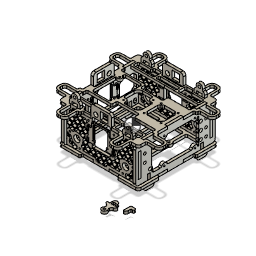
v110 (Autodesk Fusion 360 design; units mm, degrees)
Autodesk Fusion 360 part; units mm, degrees
note: some values were not read from the file. Set by a fixed rule: which sketch regions a step uses.
(part 1 of 3)
sketch "Schizzo1" plane through (0, 0, 0) normal (0, 1, 0) x (1, 0, 0)
  line L0 (-131, 140) -> (-131, 145)
  line L1 (-131, 145) -> (-111, 145)
  line L2 (-111, 140) -> (-131, 140)
  line L3 (-111, 145) -> (-111, 140)
  line L4 (-86, 145) -> (-86, 140)
  line L5 (-86, 140) -> (-71, 140)
  line L6 (-106, 147) -> (-106, 148)
  line L7 (-141, 150) -> (-108, 150)
  arc A0 (-106, 147) -> (-104, 145) centre (-104, 147) ccw
  arc A1 (-106, 148) -> (-108, 150) centre (-108, 148) ccw
  line L8 (25, 10) -> (25, 5)
  line L9 (30, 0) -> (57.5, 0)
  arc A2 (25, 5) -> (30, 0) centre (30, 5) ccw
  arc A3 (-141, 150) -> (-146, 145) centre (-141, 145) ccw
  line L10 (25, 15) -> (20, 15)
  line L11 (20, 35) -> (25, 35)
  line L12 (25, 60) -> (20, 60)
  line L13 (20, 60) -> (20, 75)
  line L14 (25, 10) -> (25, 15)
  line L15 (25, 35) -> (25, 60)
  line L16 (-141, 90) -> (-136, 90)
  line L17 (-136, 90) -> (-136, 75)
  line L18 (-143, 110) -> (-144, 110)
  line L19 (-146, 112) -> (-146, 145)
  arc A4 (-146, 112) -> (-144, 110) centre (-144, 112) ccw
  arc A5 (-141, 108) -> (-143, 110) centre (-143, 108) ccw
  line L20 (-141, 115) -> (-136, 115)
  line L21 (-136, 115) -> (-136, 135)
  line L22 (-136, 135) -> (-141, 135)
  line L23 (-141, 135) -> (-141, 115)
  arc A6 (-108, 0) -> (-106, 2) centre (-108, 2) ccw
  line L24 (-106, 3) -> (-106, 2)
  arc A7 (-104, 5) -> (-106, 3) centre (-104, 3) ccw
  line L25 (-86, 5) -> (-86, 10)
  line L26 (-86, 10) -> (-71, 10)
  line L27 (-136, 60) -> (-136, 75)
  line L28 (-141, 60) -> (-136, 60)
  arc A8 (-143, 40) -> (-141, 42) centre (-143, 42) ccw
  line L29 (-143, 40) -> (-144, 40)
  arc A9 (-144, 40) -> (-146, 38) centre (-144, 38) ccw
  line L30 (-146, 38) -> (-146, 5)
  arc A10 (-146, 5) -> (-141, 0) centre (-141, 5) ccw
  line L31 (-141, 0) -> (-108, 0)
  line L32 (-111, 10) -> (-131, 10)
  line L33 (-131, 10) -> (-131, 5)
  line L34 (-111, 5) -> (-111, 10)
  line L35 (-131, 5) -> (-111, 5)
  line L36 (-141, 15) -> (-141, 35)
  line L37 (-141, 35) -> (-136, 35)
  line L38 (-136, 15) -> (-141, 15)
  line L39 (-136, 35) -> (-136, 15)
  arc A11 (1, 110) -> (-1, 108) centre (1, 108) ccw
  line L40 (1, 110) -> (2, 110)
  arc A12 (2, 110) -> (4, 112) centre (2, 112) ccw
  line L41 (4, 112) -> (4, 145)
  arc A13 (4, 145) -> (-1, 150) centre (-1, 145) ccw
  line L42 (-1, 150) -> (-34, 150)
  arc A14 (-34, 150) -> (-36, 148) centre (-34, 148) ccw
  line L43 (-36, 147) -> (-36, 148)
  arc A15 (-38, 145) -> (-36, 147) centre (-38, 147) ccw
  line L44 (-56, 145) -> (-56, 140)
  line L45 (-56, 140) -> (-71, 140)
  line L46 (-31, 140) -> (-11, 140)
  line L47 (-11, 140) -> (-11, 145)
  line L48 (-31, 145) -> (-31, 140)
  line L49 (-11, 145) -> (-31, 145)
  line L50 (-1, 135) -> (-1, 115)
  line L51 (-1, 115) -> (-6, 115)
  line L52 (-6, 135) -> (-1, 135)
  line L53 (-6, 115) -> (-6, 135)
  line L54 (-1, 90) -> (-6, 90)
  line L55 (-6, 90) -> (-6, 75)
  line L56 (-1, 60) -> (-6, 60)
  line L57 (-6, 60) -> (-6, 75)
  line L58 (-56, 5) -> (-56, 10)
  line L59 (-56, 10) -> (-71, 10)
  arc A16 (-1, 42) -> (1, 40) centre (1, 42) ccw
  line L60 (1, 40) -> (2, 40)
  arc A17 (4, 38) -> (2, 40) centre (2, 38) ccw
  line L61 (4, 38) -> (4, 5)
  arc A18 (-1, 0) -> (4, 5) centre (-1, 5) ccw
  line L62 (-1, 0) -> (-34, 0)
  arc A19 (-36, 2) -> (-34, 0) centre (-34, 2) ccw
  line L63 (-36, 3) -> (-36, 2)
  arc A20 (-36, 3) -> (-38, 5) centre (-38, 3) ccw
  line L64 (-11, 10) -> (-11, 5)
  line L65 (-11, 5) -> (-31, 5)
  line L66 (-31, 10) -> (-11, 10)
  line L67 (-31, 5) -> (-31, 10)
  line L68 (-1, 15) -> (-1, 35)
  line L69 (-1, 35) -> (-6, 35)
  line L70 (-6, 15) -> (-1, 15)
  line L71 (-6, 35) -> (-6, 15)
  line L72 (-231.9997, 2.9999) -> (-231.9997, 2.0006)
  line L73 (-192, 38) -> (-192, 37.0001)
  line L74 (-307, 5) -> (-307, 10)
  line L75 (-197, 60) -> (-202, 60)
  arc A21 (-300, 5) -> (-302, 3) centre (-300, 3) ccw
  arc A22 (-304, 0) -> (-302, 2) centre (-304, 2) ccw
  arc A23 (-197, -0.0001) -> (-192, 4.9999) centre (-197, 4.9999) ccw
  arc A24 (-197, 42) -> (-195, 40) centre (-195, 42) ccw
  arc A25 (-342.0001, 5) -> (-337, 0) centre (-337, 5) ccw
  line L76 (-302, 3) -> (-302, 2)
  line L77 (-195, 40) -> (-194, 40)
  arc A26 (-340, 40) -> (-342, 38) centre (-340, 38) ccw
  arc A27 (-192, 38) -> (-194, 40) centre (-194, 38) ccw
  line L78 (-339, 40) -> (-340, 40)
  line L79 (-202, 60) -> (-202, 75)
  arc A28 (-339, 40) -> (-337, 42) centre (-339, 42) ccw
  arc A29 (-231.9997, 2.9999) -> (-233.9999, 5.0001) centre (-233.9999, 2.9999) ccw
  arc A30 (-231.9997, 2.0006) -> (-229.999, -0.0001) centre (-229.999, 2.0006) ccw
  line L80 (85, 0) -> (57.5, 0)
  arc A31 (85, 0) -> (90, 5) centre (85, 5) ccw
  line L81 (90, 35) -> (90, 60)
  line L82 (90, 60) -> (95, 60)
  line L83 (95, 60) -> (95, 75)
  line L84 (20, 115) -> (25, 115)
  line L85 (25, 115) -> (25, 90)
  line L86 (25, 90) -> (20, 90)
  line L87 (20, 90) -> (20, 75)
  line L88 (25, 140) -> (25, 145)
  line L89 (30, 150) -> (57.5, 150)
  arc A32 (30, 150) -> (25, 145) centre (30, 145) ccw
  line L90 (25, 135) -> (20, 135)
  line L91 (25, 140) -> (25, 135)
  line L92 (57.5, 140) -> (35, 140)
  line L93 (35, 145) -> (35, 140)
  line L94 (57.5, 145) -> (35, 145)
  line L95 (80, 145) -> (80, 140)
  line L96 (80, 140) -> (57.5, 140)
  line L97 (57.5, 145) -> (80, 145)
  arc A33 (90, 145) -> (85, 150) centre (85, 145) ccw
  line L98 (85, 150) -> (57.5, 150)
  line L99 (90, 90) -> (95, 90)
  line L100 (95, 90) -> (95, 75)
  line L101 (-280.5, -113.5) -> (-265.5, -113.5)
  line L102 (-250.5, -113.5) -> (-265.5, -113.5)
  line L103 (-305.5, -113.5) -> (-305.5, -118.5)
  line L104 (-195.5, -98.5) -> (-200.5, -98.5)
  line L105 (-225.5, -43.5) -> (-246, -43.5)
  line L106 (-340.5, -103.5) -> (-340.5, -76)
  line L107 (-251, -18.5) -> (-265.5, -18.5)
  line L108 (-330.5, -108.5) -> (-335.5, -108.5)
  line L109 (-305.5, -38.5) -> (-305.5, -43.5)
  line L110 (-280, -18.5) -> (-265.5, -18.5)
  line L111 (-225.5, -108.5) -> (-250.5, -108.5)
  arc A34 (-340.5, -103.5) -> (-335.5, -108.5) centre (-335.5, -103.5) ccw
  line L112 (-285, -43.5) -> (-285, -23.5)
  line L113 (-330.5, -43.5) -> (-325.5, -43.5)
  line L114 (-305.5, -108.5) -> (-280.5, -108.5)
  line L115 (-325.5, -43.5) -> (-325.5, -38.5)
  line L116 (-330.5, -43.5) -> (-335.5, -43.5)
  line L117 (-305.5, -113.5) -> (-305.5, -108.5)
  line L118 (-200.5, -43.5) -> (-195.5, -43.5)
  line L119 (-195.5, -53.5) -> (-200.5, -53.5)
  line L120 (-589.5, -1.5) -> (-589.5, -1.5)
  line L121 (-320.5, -123.5) -> (-310.5, -123.5)
  arc A35 (-310.5, -123.5) -> (-305.5, -118.5) centre (-310.5, -118.5) ccw
  arc A36 (-325.5, -118.5) -> (-320.5, -123.5) centre (-320.5, -118.5) ccw
  line L122 (-195.5, -76) -> (-195.5, -98.5)
  arc A37 (-335.5, -43.5) -> (-340.5, -48.5) centre (-335.5, -48.5) ccw
  line L123 (-200.5, -108.5) -> (-195.5, -108.5)
  line L124 (-200.5, -43.5) -> (-205.5, -43.5)
  line L125 (-330.5, -108.5) -> (-325.5, -108.5)
  line L126 (-305.5, -43.5) -> (-285, -43.5)
  line L127 (-190.5, -48.5) -> (-190.5, -76)
  line L128 (-225.5, -38.5) -> (-225.5, -43.5)
  line L129 (-200.5, -108.5) -> (-205.5, -108.5)
  line L130 (-340.5, -48.5) -> (-340.5, -76)
  line L131 (-246, -43.5) -> (-246, -23.5)
  arc A38 (-190.5, -48.5) -> (-195.5, -43.5) centre (-195.5, -48.5) ccw
  line L132 (-195.5, -76) -> (-195.5, -53.5)
  line L133 (-190.5, -103.5) -> (-190.5, -76)
  line L134 (-205.5, -43.5) -> (-205.5, -38.5)
  line L135 (-280.5, -108.5) -> (-280.5, -113.5)
  line L136 (-250.5, -108.5) -> (-250.5, -113.5)
  arc A39 (-195.5, -108.5) -> (-190.5, -103.5) centre (-195.5, -103.5) ccw
  arc A40 (-280, -18.5) -> (-285, -23.5) centre (-280, -23.5) ccw
  arc A41 (-246, -23.5) -> (-251, -18.5) centre (-251, -23.5) ccw
  circle A42 centre (-252.9, 89.1) radius 1.25
  circle A43 centre (-281.1, 60.9) radius 1.25
  line L137 (-252.9, 84.1) -> (-250.5, 84.1)
  line L138 (-257.9, 89.1) -> (-257.9, 91.5)
  line L139 (-281.1, 65.9) -> (-283.5, 65.9)
  line L140 (-276.1, 60.9) -> (-276.1, 58.5)
  arc A44 (-257.9, 89.1) -> (-252.9, 84.1) centre (-252.9, 89.1) ccw
  arc A45 (-276.1, 60.9) -> (-281.1, 65.9) centre (-281.1, 60.9) ccw
  arc A46 (-248, 81.6) -> (-250.5, 84.1) centre (-250.5, 81.6) ccw
  arc A47 (-257.9, 91.5) -> (-260.4, 94) centre (-260.4, 91.5) ccw
  arc A48 (-286, 68.4) -> (-283.5, 65.9) centre (-283.5, 68.4) ccw
  arc A49 (-276.1, 58.5) -> (-273.6, 56) centre (-273.6, 58.5) ccw
  line L141 (-31, 140) -> (-25, 140)
  line L142 (-337, 42) -> (-337, 55.5)
  line L143 (-300, 5) -> (-286.5, 5)
  line L144 (-247.5, 5.0001) -> (-233.9999, 5.0001)
  circle A50 centre (33, 54) radius 1.5
  circle A51 centre (33, 112) radius 1.5
  circle A52 centre (-115.5198, -118.5231) radius 1.5
  circle A53 centre (-134.2581, -99.7848) radius 1.5
  circle A54 centre (-120.8585, -105.1234) radius 6
  circle A55 centre (-98.9028, -64.4294) radius 1.5
  line L145 (-82.3205, -124) -> (-80, -124)
  line L146 (-85, -121) -> (-85, -122)
  line L147 (-132, -119) -> (-133, -119)
  line L148 (-135, -117) -> (-135, -116)
  line L149 (-130, -61) -> (-130, -62)
  line L150 (-120, -62) -> (-120, -61)
  line L151 (-80, -124) -> (-77.6795, -124)
  line L152 (-75, -114) -> (-79.3301, -116.5)
  line L153 (-79.3301, -116.5) -> (-79.3301, -121.5)
  line L154 (-79.3301, -121.5) -> (-75, -124)
  arc A56 (-85, -121) -> (-87, -119) centre (-87, -121) ccw
  arc A57 (-85, -122) -> (-84.2458, -123.5646) centre (-83, -122) ccw
  arc A58 (-135, -117) -> (-133, -119) centre (-133, -117) ccw
  arc A59 (-135, -116) -> (-135.7542, -114.4354) centre (-137, -116) ccw
  arc A60 (-130.6699, -119.5064) -> (-132, -119) centre (-132, -121) ccw
  arc A61 (-128, -59) -> (-130, -61) centre (-128, -61) ccw
  arc A62 (-120, -61) -> (-122, -59) centre (-122, -61) ccw
  arc A63 (-103.7753, -65.5513) -> (-105.7243, -64) centre (-105.7243, -66) ccw
  line L155 (-75, -114) -> (-79.3301, -116.5)
  line L156 (-79.3301, -116.5) -> (-79.3301, -121.5)
  line L157 (-79.3301, -121.5) -> (-75, -124)
  arc A64 (-120.6699, -117.2162) -> (-122.2488, -116.0352) centre (-122.5016, -118.0192) ccw
  arc A65 (-130.5673, -96.4116) -> (-127.8245, -96.6102) centre (-129.091, -95.0624) ccw
  arc A66 (-112.3453, -112.0894) -> (-112.7588, -113.747) centre (-110.7974, -113.356) ccw
  line L158 (-84.2458, -123.5646) -> (-80.6699, -121.5)
  line L159 (-80.6699, -121.5) -> (-80.6699, -116.5)
  line L160 (-80.6699, -116.5) -> (-85, -114)
  line L161 (-85, -114) -> (-89.3301, -116.5)
  line L162 (-89.3301, -116.5) -> (-89.3301, -119)
  line L163 (-90.6699, -119) -> (-90.6699, -116.5)
  line L164 (-90.6699, -116.5) -> (-95, -114)
  line L165 (-95, -114) -> (-99.3301, -116.5)
  line L166 (-99.3301, -116.5) -> (-99.3301, -119)
  line L167 (-126.72, -114.993) -> (-129.3301, -116.5)
  line L168 (-129.3301, -116.5) -> (-129.3301, -121.5)
  line L169 (-129.3301, -121.5) -> (-125, -124)
  line L170 (-125, -124) -> (-120.6699, -121.5)
  line L171 (-120.6699, -121.5) -> (-120.6699, -117.2162)
  line L172 (-130.6699, -116.5) -> (-135, -114)
  line L173 (-80, -115.3397) -> (-75.6699, -112.8397)
  line L174 (-75.6699, -112.8397) -> (-75.6699, -107.8397)
  line L175 (-75.6699, -107.8397) -> (-77.9904, -106.5)
  line L176 (-82.0096, -106.5) -> (-84.3301, -107.8398)
  line L177 (-84.3301, -107.8398) -> (-84.3301, -112.8398)
  line L178 (-84.3301, -112.8398) -> (-80, -115.3397)
  line L179 (-85.6699, -112.8397) -> (-85.6699, -107.8397)
  line L180 (-85.6699, -107.8397) -> (-87.9002, -106.5521)
  line L181 (-92.1651, -106.5898) -> (-94.3301, -107.8398)
  line L182 (-94.3301, -107.8398) -> (-94.3301, -112.8398)
  line L183 (-94.3301, -112.8398) -> (-90, -115.3397)
  line L184 (-90, -115.3397) -> (-85.6699, -112.8397)
  line L185 (-75.6699, -112.8397) -> (-75.6699, -107.8397)
  line L186 (-75.6699, -107.8397) -> (-77.9904, -106.5)
  line L187 (-82.0096, -106.5) -> (-84.3301, -107.8398)
  line L188 (-84.3301, -107.8398) -> (-84.3301, -112.8398)
  line L189 (-84.3301, -112.8398) -> (-80, -115.3397)
  line L190 (-80, -115.3397) -> (-75.6699, -112.8397)
  line L191 (-105.6699, -107.8397) -> (-109.8624, -105.4192)
  line L192 (-112.7588, -113.747) -> (-110, -115.3397)
  line L193 (-110, -115.3397) -> (-105.6699, -112.8397)
  line L194 (-105.6699, -112.8397) -> (-105.6699, -107.8397)
  line L195 (-100, -115.3397) -> (-95.6699, -112.8397)
  line L196 (-95.6699, -112.8397) -> (-95.6699, -107.8397)
  line L197 (-95.6699, -107.8397) -> (-100, -105.3397)
  line L198 (-100, -105.3397) -> (-104.3301, -107.8398)
  line L199 (-104.3301, -112.8398) -> (-100, -115.3397)
  line L200 (-104.3301, -107.8398) -> (-104.3301, -112.8398)
  line L201 (-130, -115.3397) -> (-127.4968, -113.8945)
  line L202 (-131.7929, -106.3749) -> (-134.3301, -107.8398)
  line L203 (-134.3301, -112.8398) -> (-130, -115.3397)
  line L204 (-134.3301, -107.8398) -> (-134.3301, -112.8398)
  line L205 (-80, -122.6603) -> (-82.3205, -124)
  line L206 (-77.6795, -124) -> (-80, -122.6603)
  line L207 (-100.6699, -99.1795) -> (-105, -96.6795)
  line L208 (-105, -96.6795) -> (-109.3301, -99.1795)
  line L209 (-109.3301, -99.1795) -> (-109.3301, -104.1795)
  line L210 (-109.3301, -104.1795) -> (-105, -106.6795)
  line L211 (-100.6699, -104.1795) -> (-100.6699, -99.1795)
  line L212 (-105, -106.6795) -> (-100.6699, -104.1795)
  line L213 (-135, -106.6795) -> (-132.4803, -105.2248)
  line L214 (-139.3301, -103) -> (-139.3301, -104.1795)
  line L215 (-139.3301, -104.1795) -> (-135, -106.6795)
  line L216 (-105.6699, -90.5192) -> (-110, -88.0192)
  line L217 (-110, -88.0192) -> (-114.3301, -90.5192)
  line L218 (-114.3301, -90.5192) -> (-114.3301, -95.5192)
  line L219 (-114.3301, -95.5192) -> (-110, -98.0192)
  line L220 (-110, -98.0192) -> (-105.6699, -95.5192)
  line L221 (-105.6699, -95.5192) -> (-105.6699, -90.5192)
  line L222 (-125.6699, -90.5192) -> (-130, -88.0192)
  line L223 (-130, -88.0192) -> (-134.3301, -90.5192)
  line L224 (-134.3301, -90.5192) -> (-134.3301, -94.7853)
  line L225 (-125.6699, -95.2315) -> (-125.6699, -90.5192)
  line L226 (-115.6699, -95.424) -> (-115.6699, -90.5192)
  line L227 (-115.6699, -90.5192) -> (-120, -88.0192)
  line L228 (-120, -88.0192) -> (-124.3301, -90.5192)
  line L229 (-124.3301, -90.5192) -> (-124.3301, -94.6856)
  line L230 (-140, -98.0192) -> (-138.5149, -97.1618)
  line L231 (-135.6699, -94.9882) -> (-135.6699, -90.5192)
  line L232 (-135.6699, -90.5192) -> (-140, -88.0192)
  line L233 (-100.6699, -81.859) -> (-105, -79.359)
  line L234 (-105, -79.359) -> (-109.3301, -81.859)
  line L235 (-109.3301, -81.859) -> (-109.3301, -86.859)
  line L236 (-109.3301, -86.859) -> (-105, -89.359)
  line L237 (-100.6699, -86.859) -> (-100.6699, -81.859)
  line L238 (-105, -89.359) -> (-100.6699, -86.859)
  line L239 (-110.6699, -86.859) -> (-110.6699, -81.859)
  line L240 (-110.6699, -81.859) -> (-115, -79.359)
  line L241 (-115, -79.359) -> (-119.3301, -81.859)
  line L242 (-119.3301, -81.859) -> (-119.3301, -86.859)
  line L243 (-119.3301, -86.859) -> (-115, -89.359)
  line L244 (-115, -89.359) -> (-110.6699, -86.859)
  line L245 (-120.6699, -81.859) -> (-125, -79.359)
  line L246 (-125, -79.359) -> (-129.3301, -81.859)
  line L247 (-129.3301, -81.859) -> (-129.3301, -86.859)
  line L248 (-129.3301, -86.859) -> (-125, -89.359)
  line L249 (-120.6699, -86.859) -> (-120.6699, -81.859)
  line L250 (-125, -89.359) -> (-120.6699, -86.859)
  line L251 (-130.6699, -86.859) -> (-130.6699, -81.859)
  line L252 (-130.6699, -81.859) -> (-135, -79.359)
  line L253 (-135, -79.359) -> (-139.3301, -81.859)
  line L254 (-139.3301, -81.859) -> (-139.3301, -86.859)
  line L255 (-139.3301, -86.859) -> (-135, -89.359)
  line L256 (-135, -89.359) -> (-130.6699, -86.859)
  line L257 (-134.3301, -73.1987) -> (-134.3301, -78.1987)
  line L258 (-134.3301, -78.1987) -> (-130, -80.6987)
  line L259 (-130, -80.6987) -> (-125.6699, -78.1987)
  line L260 (-125.6699, -78.1987) -> (-125.6699, -73.1987)
  line L261 (-125.6699, -73.1987) -> (-130, -70.6987)
  line L262 (-130, -70.6987) -> (-134.3301, -73.1987)
  line L263 (-124.3301, -78.1987) -> (-120, -80.6987)
  line L264 (-120, -80.6987) -> (-115.6699, -78.1987)
  line L265 (-115.6699, -78.1987) -> (-115.6699, -73.1987)
  line L266 (-115.6699, -73.1987) -> (-120, -70.6987)
  line L267 (-124.3301, -73.1987) -> (-124.3301, -78.1987)
  line L268 (-120, -70.6987) -> (-124.3301, -73.1987)
  line L269 (-114.3301, -78.1987) -> (-110, -80.6987)
  line L270 (-110, -80.6987) -> (-105.6699, -78.1987)
  line L271 (-105.6699, -78.1987) -> (-105.6699, -73.1987)
  line L272 (-105.6699, -73.1987) -> (-110, -70.6987)
  line L273 (-114.3301, -73.1987) -> (-114.3301, -78.1987)
  line L274 (-110, -70.6987) -> (-114.3301, -73.1987)
  line L275 (-108.3975, -64) -> (-109.3301, -64.5385)
  line L276 (-109.3301, -64.5385) -> (-109.3301, -69.5385)
  line L277 (-109.3301, -69.5385) -> (-105, -72.0385)
  line L278 (-105, -72.0385) -> (-100.6699, -69.5385)
  line L279 (-100.6699, -69.5385) -> (-100.6699, -69.1067)
  line L280 (-118.3454, -63.9699) -> (-119.3301, -64.5385)
  line L281 (-119.3301, -64.5385) -> (-119.3301, -69.5385)
  line L282 (-119.3301, -69.5385) -> (-115, -72.0385)
  line L283 (-115, -72.0385) -> (-110.6699, -69.5385)
  line L284 (-110.6699, -64.5385) -> (-111.6025, -64)
  line L285 (-110.6699, -69.5385) -> (-110.6699, -64.5385)
  line L286 (-125, -62.0385) -> (-129.3301, -64.5385)
  line L287 (-129.3301, -64.5385) -> (-129.3301, -69.5385)
  line L288 (-129.3301, -69.5385) -> (-125, -72.0385)
  line L289 (-125, -72.0385) -> (-120.6699, -69.5385)
  line L290 (-120.6699, -64.5385) -> (-125, -62.0385)
  line L291 (-120.6699, -69.5385) -> (-120.6699, -64.5385)
  line L292 (-120, -63.3782) -> (-119.6271, -63.1629)
  line L293 (-124.3301, -59) -> (-124.3301, -60.8782)
  line L294 (-124.3301, -60.8782) -> (-120, -63.3782)
  line L295 (-130.3729, -63.163) -> (-130, -63.3782)
  line L296 (-130, -63.3782) -> (-125.6699, -60.8782)
  line L297 (-125.6699, -60.8782) -> (-125.6699, -59)
  line L298 (-87, -119) -> (-89.3301, -119)
  line L299 (-90.6699, -119) -> (-99.3301, -119)
  arc A67 (-112.3453, -112.0894) -> (-109.8624, -105.4192) centre (-120.8585, -105.1234) ccw
  arc A68 (-115.6699, -95.424) -> (-124.3301, -94.6856) centre (-120.8585, -105.1234) ccw
  arc A69 (-125.6699, -95.2315) -> (-127.8245, -96.6102) centre (-120.8585, -105.1234) ccw
  arc A70 (-130.5673, -96.4116) -> (-134.3301, -94.7853) centre (-134.2581, -99.7848) ccw
  arc A71 (-135.6699, -94.9882) -> (-138.5149, -97.1618) centre (-134.2581, -99.7848) ccw
  arc A72 (-138.0873, -103) -> (-133.8982, -104.7718) centre (-134.2581, -99.7848) ccw
  arc A73 (-131.7702, -106.5138) -> (-131.7929, -106.3749) centre (-133.7542, -106.7666) ccw
  arc A74 (-132.4803, -105.2248) -> (-133.8982, -104.7718) centre (-133.7542, -106.7666) ccw
  line L300 (-140, -88.0192) -> (-140, -98.0192)
  arc A75 (-130.3729, -63.163) -> (-130, -62) centre (-132, -62) ccw
  line L301 (-122, -59) -> (-124.3301, -59)
  line L302 (-125.6699, -59) -> (-128, -59)
  arc A76 (-120, -62) -> (-119.6271, -63.1629) centre (-118, -62) ccw
  arc A77 (-118.3454, -63.9699) -> (-118, -64) centre (-118, -62) ccw
  line L303 (-118, -64) -> (-111.6025, -64)
  line L304 (-108.3975, -64) -> (-105.7243, -64)
  arc A78 (-103.7753, -65.5513) -> (-100.6699, -69.1067) centre (-98.9028, -64.4294) ccw
  line L305 (-135, -114) -> (-135.7542, -114.4354)
  line L306 (-130.6699, -116.5) -> (-130.6699, -119.5064)
  line L307 (-60, -124) -> (-35, -124)
  line L308 (-60, -124) -> (-60, -129)
  line L309 (-35, -124) -> (-35, -129)
  line L310 (-15, -129) -> (-15, -124)
  line L311 (-35, -129) -> (-15, -129)
  arc A79 (-55.5, -39) -> (-60.5, -34) centre (-60.5, -39) ccw
  line L312 (-55.5, -59) -> (-55.5, -39)
  line L313 (-35, -59) -> (-55.5, -59)
  line L314 (-35, -59) -> (-35, -54)
  line L315 (-30, -54) -> (-20, -54)
  line L316 (-15, -54) -> (-15, -59)
  line L317 (-10, -59) -> (-15, -59)
  line L318 (-10, -69) -> (-5, -69)
  line L319 (-5, -69) -> (-5, -114)
  line L320 (-15, -124) -> (-10, -124)
  line L321 (-5, -114) -> (-10, -114)
  circle A80 centre (-29.1416, -105.1234) radius 6
  circle A81 centre (-34.4802, -118.5231) radius 1.5
  circle A82 centre (-15.7419, -99.7848) radius 1.5
  line L322 (-75, -114) -> (-75, -114)
  circle A83 centre (-51.0972, -64.4294) radius 1.5
  circle A84 centre (82, 54) radius 1.5
  circle A85 centre (82, 112) radius 1.5
  circle A86 centre (-75, 75) radius 1.5
  circle A87 centre (-43, 45) radius 1.5
  arc A88 (-131, 18) -> (-128, 15) centre (-128, 18) ccw
  arc A89 (-45.5, 69.5) -> (-48.5, 72.5) centre (-48.5, 69.5) ccw
  line L323 (-11, 17.5) -> (-11, 75)
  line L324 (-13.9289, 15) -> (-13.5, 15)
  arc A90 (-40.5, 17.5) -> (-38, 15) centre (-38, 17.5) ccw
  arc A91 (-13.5, 15) -> (-11, 17.5) centre (-13.5, 17.5) ccw
  line L325 (-260.4, 94) -> (-278, 94)
  line L326 (-286, 86) -> (-286, 68.4)
  line L327 (-273.6, 56) -> (-256, 56)
  line L328 (-248, 64) -> (-248, 81.6)
  arc A92 (-278, 94) -> (-286, 86) centre (-278, 86) ccw
  arc A93 (-256, 56) -> (-248, 64) centre (-256, 64) ccw
  arc A94 (-48.5, 15) -> (-45.5, 18) centre (-48.5, 18) ccw
  arc A95 (-128, 135) -> (-131, 132) centre (-128, 132) ccw
  line L329 (-84, 18) -> (-84, 69.5)
  line L330 (-89, 18) -> (-89, 132)
  line L331 (-48.5, 15) -> (-81, 15)
  line L332 (-131, 18) -> (-131, 132)
  arc A96 (-81, 72.5) -> (-84, 69.5) centre (-81, 69.5) ccw
  arc A97 (-84, 18) -> (-81, 15) centre (-81, 18) ccw
  arc A98 (-92, 15) -> (-89, 18) centre (-92, 18) ccw
  arc A99 (-89, 132) -> (-92, 135) centre (-92, 132) ccw
  circle A100 centre (-292, 55) radius 1.5
  circle A101 centre (-322, 95) radius 1.5
  line L333 (-325.5, -38.5) -> (-305.5, -38.5)
  line L334 (-225.5, -38.5) -> (-205.5, -38.5)
  line L335 (-326, 91) -> (-326, 50)
  line L336 (-322, 46) -> (-294, 46)
  line L337 (-292, 48) -> (-292, 49.3431)
  line L338 (-322, 100.6569) -> (-322, 102)
  line L339 (-288, 59) -> (-288, 100)
  line L340 (-320, 104) -> (-292, 104)
  arc A102 (-324.4, 91.8) -> (-320.6667, 98.7712) centre (-322, 95) ccw
  arc A103 (-289.6, 58.2) -> (-293.3333, 51.2288) centre (-292, 55) ccw
  arc A104 (-326, 50) -> (-322, 46) centre (-322, 50) ccw
  arc A105 (-288, 100) -> (-292, 104) centre (-292, 100) ccw
  arc A106 (-294, 46) -> (-292, 48) centre (-294, 48) ccw
  arc A107 (-320, 104) -> (-322, 102) centre (-320, 102) ccw
  arc A108 (-289.6, 58.2) -> (-288, 59) centre (-289, 59) ccw
  arc A109 (-324.4, 91.8) -> (-326, 91) centre (-325, 91) ccw
  arc A110 (-292, 49.3431) -> (-293.3333, 51.2288) centre (-294, 49.3431) ccw
  arc A111 (-322, 100.6569) -> (-320.6667, 98.7712) centre (-320, 100.6569) ccw
  line L341 (-62.5, -38.44) -> (-76.5, -38.44)
  line L342 (-76.5, -38.44) -> (-76.5, -52.44)
  line L343 (-76.5, -52.44) -> (-62.5, -52.44)
  line L344 (-62.5, -52.44) -> (-62.5, -38.44)
  line L345 (-253, -22.94) -> (-253, -36.94)
  line L346 (-253, -36.94) -> (-267, -36.94)
  line L347 (-267, -36.94) -> (-267, -22.94)
  line L348 (-267, -22.94) -> (-253, -22.94)
  line L349 (20, 15) -> (20, 35)
  line L350 (20, 115) -> (20, 135)
  line L351 (-366, 23.0002) -> (-366, 27.0001)
  line L352 (-342, 38) -> (-342, 37.0001)
  line L353 (-342, 13.0001) -> (-342.0001, 5)
  arc A112 (-344, 35.0001) -> (-342, 37.0001) centre (-344, 37.0001) ccw
  arc A113 (-342, 13.0001) -> (-344, 15.0001) centre (-344, 13.0001) ccw
  arc A114 (-358, 35.0001) -> (-366, 27.0001) centre (-358, 27.0001) ccw
  arc A115 (-366, 23.0002) -> (-358, 15.0002) centre (-358, 23.0002) ccw
  line L354 (-307, -2) -> (-307, -15.9102)
  line L355 (-315, -23.9102) -> (-319, -23.9102)
  line L356 (-327, -15.9102) -> (-327, -2)
  line L357 (-337, 0) -> (-329, 0)
  line L358 (-305, 0) -> (-304, 0)
  arc A116 (-327, -2) -> (-329, 0) centre (-329, -2) ccw
  arc A117 (-305, 0) -> (-307, -2) centre (-305, -2) ccw
  arc A118 (-327, -15.9102) -> (-319, -23.9102) centre (-319, -15.9102) ccw
  arc A119 (-315, -23.9102) -> (-307, -15.9102) centre (-315, -15.9102) ccw
  line L359 (-227, -2.0001) -> (-227, -15.9189)
  arc A120 (-227, -15.9189) -> (-219, -23.9102) centre (-219, -15.9102) ccw
  line L360 (-219, -23.9102) -> (-215, -23.9102)
  arc A121 (-215, -23.9102) -> (-207, -15.9246) centre (-215, -15.9102) ccw
  line L361 (-207, -15.9246) -> (-207, -2.0001)
  arc A122 (-205, -0.0001) -> (-207, -2.0001) centre (-205, -2.0001) ccw
  arc A123 (-227, -2.0001) -> (-229, -0.0001) centre (-229, -2.0001) ccw
  line L362 (-197, -0.0001) -> (-205, -0.0001)
  line L363 (-229, -0.0001) -> (-229.999, -0.0001)
  arc A124 (-190, 15.0001) -> (-192, 13.0001) centre (-190, 13.0001) ccw
  arc A125 (-175.9914, 15.0002) -> (-168, 23.0002) centre (-176, 23.0002) ccw
  line L364 (-168, 23.0002) -> (-168, 27.0001)
  arc A126 (-168, 27.0001) -> (-176, 35.0001) centre (-176, 27.0001) ccw
  arc A127 (-192, 37.0001) -> (-190, 35.0001) centre (-190, 37.0001) ccw
  line L365 (-192, 4.9999) -> (-192, 13.0001)
  line L366 (33, 35) -> (33, 46.5838)
  line L367 (33, 61.4162) -> (33, 104.5838)
  arc A128 (34.875, 49.3649) -> (34.875, 58.6351) centre (33, 54) ccw
  arc A129 (33, 35) -> (38, 30) centre (38, 35) ccw
  arc A130 (34.875, 49.3649) -> (33, 46.5838) centre (36, 46.5838) ccw
  arc A131 (33, 61.4162) -> (34.875, 58.6351) centre (36, 61.4162) ccw
  arc A132 (34.875, 107.3649) -> (33, 104.5838) centre (36, 104.5838) ccw
  line L368 (82, 35) -> (82, 46.5838)
  arc A133 (82, 46.5838) -> (80.125, 49.3649) centre (79, 46.5838) ccw
  arc A134 (80.125, 58.6351) -> (80.125, 49.3649) centre (82, 54) ccw
  arc A135 (80.125, 58.6351) -> (82, 61.4162) centre (79, 61.4162) ccw
  line L369 (82, 61.4162) -> (82, 104.5838)
  arc A136 (82, 104.5838) -> (80.125, 107.3649) centre (79, 104.5838) ccw
  line L370 (33, 118) -> (33, 117.9161)
  line L371 (82, 118) -> (82, 117.9161)
  arc A137 (34.875, 107.3649) -> (33.8333, 116.9301) centre (33, 112) ccw
  arc A138 (81.1667, 116.9301) -> (80.125, 107.3649) centre (82, 112) ccw
  arc A139 (33, 117.9161) -> (33.8333, 116.9301) centre (34, 117.9161) ccw
  arc A140 (34, 119) -> (33, 118) centre (34, 118) ccw
  arc A141 (81.1667, 116.9301) -> (82, 117.9161) centre (81, 117.9161) ccw
  arc A142 (82, 118) -> (81, 119) centre (81, 118) ccw
  arc A143 (-131.7702, -106.5138) -> (-127.4968, -113.8945) centre (-120.8585, -105.1234) ccw
  arc A144 (-125.7732, -114.9644) -> (-122.2488, -116.0352) centre (-120.8585, -105.1234) ccw
  line L372 (-109.3301, -116.5) -> (-109.3301, -119)
  line L373 (-105, -114) -> (-109.3301, -116.5)
  line L374 (-100.6699, -116.5) -> (-105, -114)
  line L375 (-100.6699, -119) -> (-100.6699, -116.5)
  line L376 (-100.6699, -119) -> (-109.3301, -119)
  line L377 (-10, -98.0192) -> (-11.4851, -97.1618)
  line L378 (-70, -124) -> (-72.3205, -124)
  line L379 (-37.2412, -113.747) -> (-40, -115.3397)
  line L380 (-45, -96.6795) -> (-40.6699, -99.1795)
  arc A145 (-63, -119) -> (-65, -121) centre (-63, -121) ccw
  line L381 (-14.3301, -78.1987) -> (-14.3301, -73.4936)
  line L382 (-10, -105.3398) -> (-10, -107)
  line L383 (-35, -79.359) -> (-30.6699, -81.859)
  line L384 (-35.6699, -90.5192) -> (-35.6699, -95.5192)
  line L385 (-50, -115.3397) -> (-54.3301, -112.8397)
  line L386 (-64.3301, -112.8397) -> (-64.3301, -107.8397)
  arc A146 (-27.7512, -116.0352) -> (-29.3301, -117.2162) centre (-27.4984, -118.0192) ccw
  line L387 (-34.3301, -95.424) -> (-34.3301, -90.5192)
  line L388 (-55, -114) -> (-50.6699, -116.5)
  arc A147 (-22.5032, -113.8945) -> (-18.2298, -106.5138) centre (-29.1416, -105.1234) ccw
  arc A148 (-25.6699, -94.6856) -> (-34.3301, -95.424) centre (-29.1416, -105.1234) ccw
  line L389 (-25.6699, -90.5192) -> (-25.6699, -94.6856)
  line L390 (-45, -114) -> (-40.6699, -116.5)
  line L391 (-40.6699, -104.1795) -> (-45, -106.6795)
  line L392 (-59.3301, -119) -> (-59.3301, -116.5)
  line L393 (-44.3301, -112.8397) -> (-44.3301, -107.8397)
  line L394 (-63, -119) -> (-60.6699, -119)
  line L395 (-55.6699, -112.8398) -> (-60, -115.3397)
  arc A149 (-22.1755, -96.6102) -> (-19.4327, -96.4116) centre (-20.909, -95.0624) ccw
  line L396 (-74.3301, -112.8397) -> (-74.3301, -107.8397)
  line L397 (-65, -114) -> (-60.6699, -116.5)
  line L398 (-24.3301, -78.1987) -> (-24.3301, -73.1987)
  line L399 (-15, -72.0385) -> (-19.3301, -69.5385)
  line L400 (-60, -115.3397) -> (-64.3301, -112.8397)
  line L401 (-40.6699, -116.5) -> (-40.6699, -119)
  line L402 (-44.3301, -95.5192) -> (-44.3301, -90.5192)
  line L403 (-25, -79.359) -> (-20.6699, -81.859)
  line L404 (-44.3301, -90.5192) -> (-40, -88.0192)
  line L405 (-59.3301, -119) -> (-50.6699, -119)
  line L406 (-65.7542, -123.5646) -> (-69.3301, -121.5)
  line L407 (-20, -70.6987) -> (-15.6699, -73.1987)
  line L408 (-50.6699, -116.5) -> (-50.6699, -119)
  line L409 (-29.3301, -81.859) -> (-25, -79.359)
  line L410 (-60.6699, -116.5) -> (-60.6699, -119)
  line L411 (-70, -115.3397) -> (-74.3301, -112.8397)
  arc A150 (-16.1019, -104.7718) -> (-11.9128, -103) centre (-15.7419, -99.7848) ccw
  line L412 (-49.3301, -104.1795) -> (-49.3301, -99.1795)
  line L413 (-20.6699, -69.5385) -> (-25, -72.0385)
  line L414 (-25, -72.0385) -> (-29.3301, -69.5385)
  line L415 (-25, -124) -> (-29.3301, -121.5)
  line L416 (-55.6699, -107.8398) -> (-55.6699, -112.8398)
  line L417 (-41.6026, -64) -> (-40.6699, -64.5385)
  line L418 (-15.6699, -107.8398) -> (-15.6699, -112.8398)
  line L419 (-39.3301, -64.5385) -> (-38.3975, -64)
  line L420 (-49.3301, -99.1795) -> (-45, -96.6795)
  line L421 (-49.3301, -119) -> (-40.6699, -119)
  line L422 (-30.6699, -69.5385) -> (-35, -72.0385)
  line L423 (-65.6699, -107.8398) -> (-65.6699, -112.8398)
  line L424 (-65.6699, -107.8398) -> (-65.6699, -112.8398)
  line L425 (-39.3301, -81.859) -> (-35, -79.359)
  line L426 (-35, -72.0385) -> (-39.3301, -69.5385)
  line L427 (-14.9997, -72.0383) -> (-15, -72.0385)
  line L428 (-40.6699, -64.5385) -> (-40.6699, -69.5385)
  line L429 (-45, -106.6795) -> (-49.3301, -104.1795)
  line L430 (-39.3301, -69.5385) -> (-39.3301, -64.5385)
  line L431 (-45.6699, -112.8398) -> (-50, -115.3397)
  line L432 (-74.3301, -112.8397) -> (-74.3301, -107.8397)
  arc A151 (-27.7512, -116.0352) -> (-23.759, -114.7165) centre (-29.1416, -105.1234) ccw
  line L433 (-54.3301, -112.8397) -> (-54.3301, -107.8397)
  line L434 (-41.6026, -64) -> (-44.2757, -64)
  line L435 (-14.3301, -109.5064) -> (-14.3301, -107.8397)
  arc A152 (-49.3301, -69.1067) -> (-46.2247, -65.5513) centre (-51.0972, -64.4294) ccw
  line L436 (-40, -70.6987) -> (-35.6699, -73.1987)
  line L437 (-50, -105.3397) -> (-45.6699, -107.8398)
  line L438 (-40.6699, -99.1795) -> (-40.6699, -104.1795)
  arc A153 (-44.2757, -64) -> (-46.2247, -65.5513) centre (-44.2757, -66) ccw
  line L439 (-67.9904, -106.5) -> (-65.6699, -107.8398)
  line L440 (-10.6699, -86.859) -> (-15, -89.359)
  line L441 (-54.3301, -107.8397) -> (-50, -105.3397)
  line L442 (-30.6699, -86.859) -> (-35, -89.359)
  line L443 (-10.6699, -104.1795) -> (-15, -106.6795)
  arc A154 (-22.1755, -96.6102) -> (-24.3301, -95.2315) centre (-29.1416, -105.1234) ccw
  line L444 (-10, -80.6987) -> (-14.3301, -78.1987)
  line L445 (-25.6699, -78.1987) -> (-30, -80.6987)
  line L446 (-30, -63.3782) -> (-30.3729, -63.1629)
  line L447 (-70.6699, -116.5) -> (-70.6699, -121.5)
  line L448 (-19.6271, -63.163) -> (-20, -63.3782)
  line L449 (-49.3301, -86.859) -> (-49.3301, -81.859)
  line L450 (-49.3301, -81.859) -> (-45, -79.359)
  line L451 (-15.6699, -78.1987) -> (-20, -80.6987)
  arc A155 (-16.1019, -104.7718) -> (-17.5197, -105.2248) centre (-16.2458, -106.7666) ccw
  line L452 (-10.0103, -75.7973) -> (-10, -80.6987)
  line L453 (-29.3301, -69.5385) -> (-29.3301, -64.5385)
  line L454 (-14.3301, -107.8397) -> (-10, -105.3397)
  line L455 (-69.3301, -116.5) -> (-65, -114)
  line L456 (-40, -80.6987) -> (-44.3301, -78.1987)
  line L457 (-23.759, -114.7165) -> (-20.6699, -116.5)
  line L458 (-40.6699, -81.859) -> (-40.6699, -86.859)
  line L459 (-14.3301, -90.5192) -> (-10, -88.0192)
  line L460 (-75, -114) -> (-70.6699, -116.5)
  line L461 (-29.3301, -121.5) -> (-29.3301, -117.2162)
  line L462 (-75, -114) -> (-75, -114)
  arc A156 (-20, -61) -> (-22, -59) centre (-22, -61) ccw
  line L463 (-70.6699, -121.5) -> (-75, -124)
  line L464 (-20, -115.3397) -> (-22.5032, -113.8945)
  arc A157 (-18, -119) -> (-19.3301, -119.5064) centre (-18, -121) ccw
  arc A158 (-30.3729, -63.1629) -> (-30, -62) centre (-32, -62) ccw
  line L465 (-34.3301, -73.1987) -> (-30, -70.6987)
  line L466 (-24.3301, -60.8782) -> (-24.3301, -59)
  line L467 (-15.6699, -73.1987) -> (-15.6699, -78.1987)
  line L468 (-15, -106.6795) -> (-17.5197, -105.2248)
  line L469 (-65, -121) -> (-65, -122)
  arc A159 (-15, -66) -> (-17, -64) centre (-17, -66) ccw
  line L470 (-45, -79.359) -> (-40.6699, -81.859)
  line L471 (-39.3301, -86.859) -> (-39.3301, -81.859)
  line L472 (-24.3301, -95.2315) -> (-24.3301, -90.5192)
  line L473 (-10, -88.0192) -> (-10, -98.0192)
  line L474 (-20, -63.3782) -> (-24.3301, -60.8782)
  line L475 (-15, -79.359) -> (-10.6699, -81.859)
  line L476 (-70.6699, -116.5) -> (-70.6699, -121.5)
  line L477 (-44.3301, -73.1987) -> (-40, -70.6987)
  line L478 (-15, -67) -> (-15, -66)
  line L479 (-14.3301, -94.9882) -> (-14.3301, -90.5192)
  line L480 (-18, -119) -> (-17, -119)
  line L481 (-19.3301, -116.5) -> (-15, -114)
  line L482 (-10.6699, -81.859) -> (-10.6699, -86.859)
  line L483 (-25.6699, -73.1987) -> (-25.6699, -78.1987)
  arc A160 (-15.6699, -94.7853) -> (-19.4327, -96.4116) centre (-15.7419, -99.7848) ccw
  line L484 (-31.6546, -63.9699) -> (-30.6699, -64.5385)
  line L485 (-15.6699, -112.8398) -> (-20, -115.3397)
  arc A161 (-11.4851, -97.1618) -> (-14.3301, -94.9882) centre (-15.7419, -99.7848) ccw
  line L486 (-49.3301, -69.5385) -> (-49.3301, -69.1067)
  line L487 (-29.3301, -86.859) -> (-29.3301, -81.859)
  line L488 (-59.3301, -116.5) -> (-55, -114)
  line L489 (-34.3301, -90.5192) -> (-30, -88.0192)
  line L490 (-69.3301, -121.5) -> (-69.3301, -116.5)
  line L491 (-67.6795, -124) -> (-70, -124)
  line L492 (-49.3301, -119) -> (-49.3301, -116.5)
  line L493 (-45, -72.0385) -> (-49.3301, -69.5385)
  line L494 (-24.3301, -90.5192) -> (-20, -88.0192)
  line L495 (-35.6699, -95.5192) -> (-40, -98.0192)
  line L496 (-24.3301, -73.1987) -> (-20, -70.6987)
  line L497 (-30, -80.6987) -> (-34.3301, -78.1987)
  line L498 (-20, -80.6987) -> (-24.3301, -78.1987)
  line L499 (-30, -88.0192) -> (-25.6699, -90.5192)
  line L500 (-18.2071, -106.3749) -> (-15.6699, -107.8398)
  arc A162 (-37.2412, -113.747) -> (-37.6548, -112.0894) centre (-39.2026, -113.356) ccw
  line L501 (-40, -88.0192) -> (-35.6699, -90.5192)
  line L502 (-19.3301, -81.859) -> (-15, -79.359)
  line L503 (-28, -59) -> (-25.6699, -59)
  line L504 (-45.6699, -107.8398) -> (-45.6699, -112.8398)
  line L505 (-65.6699, -112.8398) -> (-70, -115.3397)
  line L506 (-20, -88.0192) -> (-15.6699, -90.5192)
  arc A163 (-18.2071, -106.3749) -> (-18.2298, -106.5138) centre (-16.2458, -106.7666) ccw
  line L507 (-19.3301, -86.859) -> (-19.3301, -81.859)
  line L508 (-40, -98.0192) -> (-44.3301, -95.5192)
  line L509 (-34.3301, -78.1987) -> (-34.3301, -73.1987)
  line L510 (-44.3301, -78.1987) -> (-44.3301, -73.1987)
  line L511 (-70, -115.3397) -> (-74.3301, -112.8397)
  line L512 (-30.6699, -81.859) -> (-30.6699, -86.859)
  line L513 (-20.6699, -81.859) -> (-20.6699, -86.859)
  line L514 (-15, -117) -> (-15, -116)
  arc A164 (-65.7542, -123.5646) -> (-65, -122) centre (-67, -122) ccw
  line L515 (-30, -70.6987) -> (-25.6699, -73.1987)
  line L516 (-44.3301, -107.8397) -> (-40.1376, -105.4192)
  line L517 (-72.3205, -124) -> (-70, -122.6603)
  line L518 (-10.6699, -103) -> (-10.6699, -104.1795)
  arc A165 (-40.1376, -105.4192) -> (-37.6548, -112.0894) centre (-29.1416, -105.1234) ccw
  line L519 (-40, -115.3397) -> (-44.3301, -112.8397)
  line L520 (-40.6699, -69.5385) -> (-45, -72.0385)
  line L521 (-15.6699, -90.5192) -> (-15.6699, -94.7853)
  line L522 (-35.6699, -73.1987) -> (-35.6699, -78.1987)
  line L523 (-67.9904, -106.5) -> (-65.6699, -107.8398)
  line L524 (-74.3301, -107.8397) -> (-72.0096, -106.5)
  line L525 (-74.3301, -107.8397) -> (-72.0096, -106.5)
  line L526 (-40.6699, -86.859) -> (-45, -89.359)
  line L527 (-20.6699, -86.859) -> (-25, -89.359)
  line L528 (-15, -89.359) -> (-19.3301, -86.859)
  line L529 (-35, -89.359) -> (-39.3301, -86.859)
  line L530 (-49.3301, -116.5) -> (-45, -114)
  line L531 (-64.3301, -107.8397) -> (-62.0096, -106.5)
  line L532 (-32, -64) -> (-38.3975, -64)
  line L533 (-35.6699, -78.1987) -> (-40, -80.6987)
  line L534 (-25.6699, -60.8782) -> (-30, -63.3782)
  line L535 (-29.3301, -64.5385) -> (-25, -62.0385)
  line L536 (-70, -122.6603) -> (-67.6795, -124)
  line L537 (-20.6699, -64.5385) -> (-20.6699, -69.5385)
  line L538 (-20.6699, -116.5) -> (-20.6699, -121.5)
  arc A166 (-28, -59) -> (-30, -61) centre (-28, -61) ccw
  arc A167 (-18.3454, -63.9699) -> (-18, -64) centre (-18, -62) ccw
  line L539 (-19.3301, -116.5) -> (-19.3301, -119.5064)
  line L540 (-30.6699, -64.5385) -> (-30.6699, -69.5385)
  line L541 (-75, -114) -> (-70.6699, -116.5)
  line L542 (-20, -61) -> (-20, -62)
  arc A168 (-32, -64) -> (-31.6546, -63.9699) centre (-32, -62) ccw
  line L543 (-19.3301, -69.5385) -> (-19.3301, -64.5385)
  arc A169 (-20, -62) -> (-19.6271, -63.163) centre (-18, -62) ccw
  line L544 (-19.3301, -64.5385) -> (-18.3454, -63.9699)
  line L545 (-24.3301, -59) -> (-22, -59)
  line L546 (-30, -62) -> (-30, -61)
  arc A170 (-17, -119) -> (-15, -117) centre (-17, -117) ccw
  line L547 (-25, -62.0385) -> (-20.6699, -64.5385)
  line L548 (-25.6699, -59) -> (-25.6699, -60.8782)
  line L549 (-70.6699, -121.5) -> (-75, -124)
  line L550 (-65.6699, -112.8398) -> (-70, -115.3397)
  line L551 (-10.6699, -69.5064) -> (-10.6699, -69.5385)
  line L552 (-17, -64) -> (-18, -64)
  line L553 (-20.6699, -121.5) -> (-25, -124)
  line L554 (-45, -89.359) -> (-49.3301, -86.859)
  line L555 (-25, -89.359) -> (-29.3301, -86.859)
  line L556 (-57.9904, -106.5) -> (-55.6699, -107.8398)
  line L557 (-138.0873, -103) -> (-139.3301, -103)
  line L558 (-11.9128, -103) -> (-10.6699, -103)
  arc A171 (-125.7732, -114.9644) -> (-126.72, -114.993) centre (-126.22, -115.8591) ccw
  line L559 (-1, 108) -> (-1, 90)
  line L560 (-1, 42) -> (-1, 60)
  line L561 (-197, 42) -> (-197, 60)
  line L562 (-35, -54) -> (-35, -49)
  line L563 (-15, -49) -> (-15, -54)
  line L564 (-30, -49) -> (-20, -49)
  line L565 (-20, -49) -> (-20, -54)
  line L566 (-20, -54) -> (-30, -54)
  line L567 (-30, -54) -> (-30, -49)
  line L568 (-120.0001, -54) -> (-120.0001, -49)
  line L569 (-120.0001, -49) -> (-130.0001, -49)
  line L570 (-120.0001, -54) -> (-130.0001, -54)
  line L571 (-130.0001, -49) -> (-130.0001, -54)
  line L572 (15, -50) -> (15, -50)
  line L573 (15, -50) -> (10, -50)
  line L574 (10, -50) -> (10, -45)
  line L575 (5, -40) -> (5, -40)
  line L576 (0, -45) -> (0, -50)
  line L577 (0, -50) -> (-5, -50)
  line L578 (-5, -50) -> (-5, -50)
  arc A172 (-5, -50) -> (-1.4897, -54.7729) centre (0, -50) ccw
  arc A173 (11.4897, -54.7729) -> (15, -50) centre (10, -50) ccw
  arc A174 (5, -40) -> (0, -45) centre (5, -45) ccw
  arc A175 (10, -45) -> (5, -40) centre (5, -45) ccw
  line L579 (-13.9289, 15) -> (-38, 15)
  line L580 (-325.5, -118.5) -> (-325.5, -108.5)
  line L581 (-305.5, -108.5) -> (-305.5, -113.5)
  line L582 (-225.5, -113.5) -> (-225.5, -118.5)
  arc A176 (-225.5, -118.5) -> (-220.5, -123.5) centre (-220.5, -118.5) ccw
  line L583 (-210.5, -123.5) -> (-220.5, -123.5)
  arc A177 (-210.5, -123.5) -> (-205.5, -118.5) centre (-210.5, -118.5) ccw
  line L584 (-205.5, -118.5) -> (-205.5, -108.5)
  line L585 (-220.5, -118.5) -> (-220.5, -113.5)
  line L586 (-210.5, -118.5) -> (-210.5, -113.5)
  line L587 (-225.5, -113.5) -> (-225.5, -108.5)
  line L588 (-220.5, -118.5) -> (-210.5, -118.5)
  line L589 (95, 134.9866) -> (99.9997, 134.9859)
  line L590 (100.0021, 134.9863) -> (99.9997, 134.9859)
  arc A178 (105.0018, 129.986) -> (100.0021, 134.9863) centre (100.0018, 129.9863) ccw
  line L591 (105.0016, 119.999) -> (105.0018, 129.986)
  arc A179 (100.0016, 114.999) -> (105.0016, 119.999) centre (100.0016, 119.999) ccw
  line L592 (100.0018, 129.9863) -> (95.0022, 129.9866)
  line L593 (100.0016, 119.999) -> (95.0018, 119.9993)
  line L594 (100.0018, 129.9863) -> (100.0016, 119.999)
  line L595 (90, 134.9873) -> (95, 134.9866)
  line L596 (100.0021, 15.0137) -> (99.9997, 15.0141)
  arc A180 (100.0021, 15.0137) -> (105.0018, 20.014) centre (100.0018, 20.0137) ccw
  line L597 (105.0016, 30.001) -> (105.0018, 20.014)
  arc A181 (105.0016, 30.001) -> (100.0016, 35.001) centre (100.0016, 30.001) ccw
  line L598 (100.0016, 35.001) -> (90, 35.0009)
  line L599 (90, 134.9873) -> (90, 145)
  line L600 (90, 90) -> (90, 115)
  line L601 (90, 115) -> (100.0016, 114.999)
  line L602 (90, 5) -> (90, 15)
  line L603 (90, 15) -> (99.9997, 15.0141)
  line L604 (95.0019, 122.4929) -> (80.0019, 122.4936)
  line L605 (80.0019, 122.4936) -> (80.002, 124.9936)
  line L606 (95.0021, 127.4929) -> (80.0021, 127.4936)
  line L607 (80.0021, 127.4936) -> (80.002, 124.9936)
  line L608 (95.0022, 129.9866) -> (95.0021, 127.4929)
  line L609 (95.0019, 122.4929) -> (95.0018, 119.9993)
  line L610 (100.0018, 20.0137) -> (100.0016, 30.001)
  line L611 (95.0022, 20.0134) -> (95.0021, 22.5071)
  line L612 (95.0021, 22.5071) -> (80.0021, 22.5064)
  line L613 (80.0021, 22.5064) -> (80.002, 25.0064)
  line L614 (100.0018, 20.0137) -> (95.0022, 20.0134)
  line L615 (95.0019, 27.5071) -> (95.0018, 30.0007)
  line L616 (95.0019, 27.5071) -> (80.0019, 27.5064)
  line L617 (80.0019, 27.5064) -> (80.002, 25.0064)
  line L618 (100.0016, 30.001) -> (95.0018, 30.0007)
  line L619 (-218, -113.5) -> (-218, -98.5)
  line L620 (-218, -98.5) -> (-215.5, -98.5)
  line L621 (-213, -113.5) -> (-213, -98.5)
  line L622 (-213, -98.5) -> (-215.5, -98.5)
  line L623 (-220.5, -113.5) -> (-218, -113.5)
  line L624 (-213, -113.5) -> (-210.5, -113.5)
  line L625 (-320.5, -118.5) -> (-320.5, -113.5)
  line L626 (-318, -113.5) -> (-320.5, -113.5)
  line L627 (-318, -98.5) -> (-315.5, -98.5)
  line L628 (-318, -113.5) -> (-318, -98.5)
  line L629 (-310.5, -113.5) -> (-313, -113.5)
  line L630 (-313, -113.5) -> (-313, -98.5)
  line L631 (-313, -98.5) -> (-315.5, -98.5)
  line L632 (-310.5, -118.5) -> (-310.5, -113.5)
  line L633 (-310.5, -118.5) -> (-320.5, -118.5)
  line L634 (5, -50) -> (2.5, -50)
  line L635 (2.5, -50) -> (2.5, -45)
  line L636 (2.5, -45) -> (7.5, -45)
  line L637 (7.5, -45) -> (7.5, -50)
  line L638 (7.5, -50) -> (5, -50)
  line L639 (25, -50) -> (25, -50)
  line L640 (30, -45) -> (30, -40)
  line L641 (30, -40) -> (33, -40)
  line L642 (35, -38) -> (35, -37)
  line L643 (33, -35) -> (27, -35)
  line L644 (25, -37) -> (25, -48.873)
  arc A182 (26.25, -49.8412) -> (30, -45) centre (25, -45) ccw
  arc A183 (33, -40) -> (35, -38) centre (33, -38) ccw
  arc A184 (35, -37) -> (33, -35) centre (33, -37) ccw
  arc A185 (27, -35) -> (25, -37) centre (27, -37) ccw
  arc A186 (25, -48.873) -> (26.25, -49.8412) centre (26, -48.873) ccw
  line L645 (-315, -19.9102) -> (-319, -19.9102)
  arc A187 (-323, -15.9098) -> (-319, -19.9102) centre (-319, -15.9102) ccw
  arc A188 (-315, -19.9102) -> (-311, -15.9102) centre (-315, -15.9102) ccw
  arc A189 (-358, 30.9999) -> (-362, 27) centre (-358, 26.9999) ccw
  line L646 (-362, 27) -> (-362, 23)
  arc A190 (-362, 23) -> (-358, 18.9999) centre (-358, 22.9999) ccw
  arc A191 (-330, 43) -> (-332, 41) centre (-330, 41) ccw
  line L647 (-332, 41) -> (-332, 37)
  arc A192 (-334, 35) -> (-332, 37) centre (-334, 37) ccw
  line L648 (-337, 35) -> (-334, 35)
  line L649 (-332, 15) -> (-337, 15)
  line L650 (-332, 23.9999) -> (-332, 15)
  arc A193 (-330, 25.9999) -> (-332, 23.9999) centre (-330, 23.9999) ccw
  line L651 (-267, 26) -> (-330, 25.9999)
  line L652 (-283, 53) -> (-267, 53)
  line L653 (-330, 43) -> (-287, 43)
  line L654 (-285, 45) -> (-285, 51)
  arc A194 (-287, 43) -> (-285, 45) centre (-287, 45) ccw
  arc A195 (-283, 53) -> (-285, 51) centre (-283, 51) ccw
  line L655 (-128, 15) -> (-92, 15)
  line L656 (-128, 135) -> (-92, 135)
  line L657 (-48.5, 72.5) -> (-69.6381, 72.5)
  line L658 (-80.3619, 72.5) -> (-81, 72.5)
  arc A196 (-46.2143, 48.8299) -> (-46.2143, 41.1701) centre (-43, 45) ccw
  arc A197 (-39.7857, 41.1701) -> (-39.7857, 48.8299) centre (-43, 45) ccw
  line L659 (-45.5, 69.5) -> (-45.5, 50.3619)
  line L660 (-45.5, 39.6381) -> (-45.5, 18)
  line L661 (-40.5, 17.5) -> (-40.5, 39.6381)
  line L662 (-40.5, 50.3619) -> (-40.5, 75)
  line L663 (-80.3619, 77.5) -> (-81, 77.5)
  arc A198 (-84, 80.5) -> (-81, 77.5) centre (-81, 80.5) ccw
  line L664 (-84, 132) -> (-84, 80.5)
  arc A199 (-81, 135) -> (-84, 132) centre (-81, 132) ccw
  line L665 (-48.5, 135) -> (-81, 135)
  arc A200 (-45.5, 132) -> (-48.5, 135) centre (-48.5, 132) ccw
  line L666 (-45.5, 110.3619) -> (-45.5, 132)
  arc A201 (-46.2143, 108.8299) -> (-46.2143, 101.1701) centre (-43, 105) ccw
  line L667 (-45.5, 80.5) -> (-45.5, 99.6381)
  arc A202 (-48.5, 77.5) -> (-45.5, 80.5) centre (-48.5, 80.5) ccw
  line L668 (-48.5, 77.5) -> (-69.6381, 77.5)
  arc A203 (-78.8299, 71.7857) -> (-71.1701, 71.7857) centre (-75, 75) ccw
  arc A204 (-71.1701, 78.2143) -> (-78.8299, 78.2143) centre (-75, 75) ccw
  arc A205 (-78.8299, 71.7857) -> (-80.3619, 72.5) centre (-80.3619, 70.5) ccw
  arc A206 (-80.3619, 77.5) -> (-78.8299, 78.2143) centre (-80.3619, 79.5) ccw
  arc A207 (-71.1701, 78.2143) -> (-69.6381, 77.5) centre (-69.6381, 79.5) ccw
  arc A208 (-69.6381, 72.5) -> (-71.1701, 71.7857) centre (-69.6381, 70.5) ccw
  arc A209 (-45.5, 99.6381) -> (-46.2143, 101.1701) centre (-47.5, 99.6381) ccw
  arc A210 (-46.2143, 108.8299) -> (-45.5, 110.3619) centre (-47.5, 110.3619) ccw
  arc A211 (-46.2143, 48.8299) -> (-45.5, 50.3619) centre (-47.5, 50.3619) ccw
  arc A212 (-45.5, 39.6381) -> (-46.2143, 41.1701) centre (-47.5, 39.6381) ccw
  arc A213 (-39.7857, 41.1701) -> (-40.5, 39.6381) centre (-38.5, 39.6381) ccw
  arc A214 (-40.5, 50.3619) -> (-39.7857, 48.8299) centre (-38.5, 50.3619) ccw
  line L669 (-11, 132.5) -> (-11, 75)
  arc A215 (-11, 132.5) -> (-13.5, 135) centre (-13.5, 132.5) ccw
  line L670 (-13.9289, 135) -> (-13.5, 135)
  line L671 (-13.9289, 135) -> (-38, 135)
  arc A216 (-38, 135) -> (-40.5, 132.5) centre (-38, 132.5) ccw
  line L672 (-40.5, 132.5) -> (-40.5, 110.3619)
  arc A217 (-40.5, 110.3619) -> (-39.7857, 108.8299) centre (-38.5, 110.3619) ccw
  arc A218 (-39.7857, 101.1701) -> (-39.7857, 108.8299) centre (-43, 105) ccw
  arc A219 (-39.7857, 101.1701) -> (-40.5, 99.6381) centre (-38.5, 99.6381) ccw
  line L673 (-40.5, 99.6381) -> (-40.5, 75)
  circle A220 centre (-43, 105) radius 1.5
  arc A221 (1.9074, -58.4876) -> (1.899, -58.4495) centre (-5, -60) ccw
  arc A222 (8.101, -58.4495) -> (8.0926, -58.4876) centre (15, -60) ccw
  arc A223 (0.4822, -67.1423) -> (9.5178, -67.1423) centre (5, -65) ccw
  arc A224 (1.899, -58.4495) -> (-1.4897, -54.7729) centre (-2.9793, -59.5459) ccw
  arc A225 (11.4897, -54.7729) -> (8.101, -58.4495) centre (12.9793, -59.5459) ccw
  circle A226 centre (5, -65) radius 2
  arc A227 (1.1111, -61.8573) -> (8.8889, -61.8573) centre (5, -65) ccw
  arc A228 (1.1111, -61.8573) -> (1.9074, -58.4876) centre (-2, -59.3431) ccw
  arc A229 (8.0926, -58.4876) -> (8.8889, -61.8573) centre (12, -59.3431) ccw
  line L674 (-323, -15.9098) -> (-322.9979, 2.9998)
  line L675 (-311, -15.9102) -> (-311, 3)
  line L676 (-327, 5) -> (-324.9979, 5)
  line L677 (-309, 5) -> (-307, 5)
  arc A230 (-322.9979, 2.9998) -> (-324.9979, 5) centre (-324.9979, 3) ccw
  arc A231 (-309, 5) -> (-311, 3) centre (-309, 3) ccw
  line L678 (-337, 15) -> (-337, 16.9999)
  line L679 (-337, 33) -> (-337, 35)
  arc A232 (-339, 31) -> (-337, 33) centre (-339, 33) ccw
  arc A233 (-337, 16.9999) -> (-339, 18.9999) centre (-339, 16.9999) ccw
  line L680 (-267, 26) -> (-204, 25.9999)
  arc A234 (-202, 23.9999) -> (-204, 25.9999) centre (-204, 23.9999) ccw
  line L681 (-202, 23.9999) -> (-202, 15)
  line L682 (-202, 15) -> (-197, 15)
  line L683 (-197, 15) -> (-197, 16.9999)
  arc A235 (-195, 18.9999) -> (-197, 16.9999) centre (-195, 16.9999) ccw
  arc A236 (-176, 18.9999) -> (-172, 23) centre (-176, 22.9999) ccw
  line L684 (-172, 27) -> (-172, 23)
  arc A237 (-172, 27) -> (-176, 30.9999) centre (-176, 26.9999) ccw
  arc A238 (-197, 33) -> (-195, 31) centre (-195, 33) ccw
  line L685 (-197, 33) -> (-197, 35)
  line L686 (-197, 35) -> (-200, 35)
  arc A239 (-202, 37) -> (-200, 35) centre (-200, 37) ccw
  line L687 (-202, 41) -> (-202, 37)
  arc A240 (-202, 41) -> (-204, 43) centre (-204, 41) ccw
  line L688 (-204, 43) -> (-241, 43)
  arc A241 (-243, 45) -> (-241, 43) centre (-241, 45) ccw
  line L689 (-243, 45) -> (-243, 51)
  arc A242 (-243, 51) -> (-245, 53) centre (-245, 51) ccw
  line L690 (-245, 53) -> (-267, 53)
  line L691 (-267, 124) -> (-204, 124.0001)
  arc A243 (-204, 124.0001) -> (-202, 126.0001) centre (-204, 126.0001) ccw
  line L692 (-202, 126.0001) -> (-202, 135)
  line L693 (-202, 135) -> (-197, 135)
  line L694 (-197, 135) -> (-197, 133.0001)
  arc A244 (-197, 133.0001) -> (-195, 131.0001) centre (-195, 133.0001) ccw
  arc A245 (-172, 127) -> (-176, 131.0001) centre (-176, 127.0001) ccw
  line L695 (-172, 123) -> (-172, 127)
  arc A246 (-176, 119.0001) -> (-172, 123) centre (-176, 123.0001) ccw
  arc A247 (-195, 119) -> (-197, 117) centre (-195, 117) ccw
  line L696 (-197, 117) -> (-197, 115)
  line L697 (-197, 115) -> (-200, 115)
  arc A248 (-200, 115) -> (-202, 113) centre (-200, 113) ccw